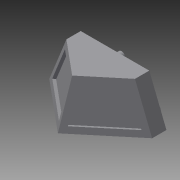
# Autodesk Inventor part: Cow Catcher
Saved by Autodesk Inventor 2015 (Build 190159000, 159)
## iProperties
Created: 2018-03-27
Part Number: Cow Catcher
Material: Generic
Document SubType Name: Modeling
Designer: Administrator
Density: 1 g/cm^3
Appearance: Default
Author: Administrator
Autodesk Inventor part; units mm, degrees
ref_plane "YZ Plane" through (0, 0, 0) normal (1, 0, 0) x (0, 1, 0)
ref_plane "XZ Plane" through (0, 0, 0) normal (0, 1, 0) x (-1, 0, 0)
ref_plane "XY Plane" through (0, 0, 0) normal (0, 0, 1) x (1, 0, 0)
sketch "Sketch1" plane through (0, 0, 0) normal (0, 1, 0) x (-1, 0, 0)
  line L0 (-3.711, -25.8637) -> (-3.711, -32.2137)
  line L1 (-3.711, -32.2137) -> (-49.431, -32.2137)
  line L2 (-49.431, -32.2137) -> (-49.431, -25.8637)
  line L3 (-3.711, -25.8637) -> (-26.571, -6.8137)
  line L4 (-26.571, -6.8137) -> (-49.431, -25.8637)
  point P0 (0, 0)
  dimension "d0" = 6.35
  dimension "d1" = 6.35
  dimension "d2" = 45.72
  dimension "d3" = 22.86
  dimension "d4" = 22.86
  dimension "d5" = 25.4
  constraints: 10 end point, 2 perpendicular
  measures "d0" distance of L0.start L0.end
  measures "d1" distance of L1.end L2.end
  measures "d2" distance of L0.end L1.end
  measures "d3" horizontal distance of L3.end L2.end
  measures "d4" horizontal distance of L0.start L3.end
  measures "d5" distance from line of L3.end L1
ref_plane "Work Plane2" through (0, 19.05, 0) normal (0, 1, 0) x (1, 0, 0)
sketch "Sketch2" plane through (0, 19.05, 0) normal (0, 1, 0) x (1, 0, 0)
  line L0 (41.811, 32.2137) -> (11.331, 32.2137)
  line L1 (11.331, 32.2137) -> (11.331, 25.8637)
  line L2 (11.331, 25.8637) -> (26.571, 13.1637)
  line L3 (26.571, 13.1637) -> (41.811, 25.8637)
  line L4 (41.811, 25.8637) -> (41.811, 32.2137)
  point P0 (0, 0)
  point P1 (26.571, 6.8137)
  dimension "d8" = 6.35
  dimension "d9" = 6.35
  dimension "d10" = 15.24
  dimension "d11" = 15.24
  dimension "d12" = 30.48
  dimension "d15" = 0
  constraints: 10 end point, 1 perpendicular, 1 vertical
  measures "d8" distance of L0.end L1.end
  measures "d9" distance of L3.end L0.start
  measures "d10" horizontal distance of L2.end L3.end
  measures "d11" horizontal distance of L1.end L2.end
  measures "d12" distance of L0.start L0.end
  measures "d15" horizontal distance of point (26.571, 6.814) L2.end
loft "Loft1" add profiles "Sketch1", "Sketch2"
shell "Shell1" thickness 2.54 removed faces 1 at (26.571, 0, -23.7471)
sketch "Sketch4" plane through (26.571, 0, -6.8137) normal (0.6201737, 0.2480695, 0.7442084) x (0.7682213, 0, -0.6401844)
  line L0 (0, 0) -> (4.0652, 19.6647) projected
  line L1 (29.7571, 0) -> (23.9032, 19.6647) projected
  line L2 (29.7571, 0) -> (0, 0) projected
  line L3 (23.9032, 19.6647) -> (4.0652, 19.6647) projected
  line L4 (3.1188, 2.54) -> (6.1338, 17.1247)
  line L5 (6.1338, 17.1247) -> (22.0092, 17.1247)
  line L6 (22.0092, 17.1247) -> (26.3508, 2.54)
  line L7 (26.3508, 2.54) -> (3.1188, 2.54)
  point P0 (-24.7744, 2.9212)
  dimension "d21" = 2.54
  dimension "d22" = 2.54
  dimension "d23" = 2.54
  dimension "d24" = 2.54
  constraints: 8 end point, 5 parallel, 1 horizontal
  measures "d21" distance between parallel lines of L2 L7
  measures "d22" distance between parallel lines of L0 L4
  measures "d23" distance between parallel lines of L3 L5
  measures "d24" distance between parallel lines of L1 L6
extrude "Extrusion2" cut sketch "Sketch4" against normal blind 1.27 contours L4 L5 L6 L7
sketch "Sketch5" plane through (3.711, 0, -25.8637) normal (-0.6201737, 0.2480695, 0.7442084) x (0.7682213, 0, 0.6401844)
  line L0 (29.7571, 0) -> (0, 0)
  line L1 (24.1888, 19.6583) -> (4.3507, 19.6583)
  line L2 (3.4063, 2.54) -> (7.746, 17.1183)
  line L3 (7.746, 17.1183) -> (23.6246, 17.1183)
  line L4 (23.6246, 17.1183) -> (26.6383, 2.54)
  line L5 (26.6383, 2.54) -> (3.4063, 2.54)
  line L6 (0, 0) -> (5.8538, 19.6647) projected
  line L7 (29.7571, 0) -> (25.6919, 19.6647) projected
  point P0 (13.7067, -5.5182)
  point P1 (-24.7744, 2.9212)
  dimension "d27" = 2.54
  dimension "d29" = 2.54
  dimension "d32" = 2.54
  dimension "d34" = 2.54
  constraints: 12 end point, 4 parallel, 1 horizontal
  measures "d27" distance between parallel lines of L0 L5
  measures "d29" distance between parallel lines of L1 L3
  measures "d32" distance between parallel lines of L6 L2
  measures "d34" distance between parallel lines of L7 L4
extrude "Extrusion3" cut sketch "Sketch5" against normal blind 1.27
sketch "Sketch6" plane through (49.431, 0, -32.2137) normal (0, 0, -1) x (-1, 0, 0)
  circle A0 centre (6.985, 3.175) radius 1.5875
  circle A1 centre (22.86, 15.875) radius 1.5875
  circle A2 centre (38.735, 3.175) radius 1.5875
  line L0 (0, 0) -> (7.62, 19.05) projected
  line L1 (45.72, 0) -> (0, 0) projected
  line L2 (45.72, 0) -> (38.1, 19.05) projected
  line L3 (38.1, 19.05) -> (7.62, 19.05) projected
  point P0 (49.431, 0)
  dimension "d37" = 6.985
  dimension "d38" = 6.985
  dimension "d39" = 3.175
  dimension "d40" = 3.175
  dimension "d41" = 3.175
  dimension "d42" = 22.86
  dimension "d43" = 3.175
  dimension "d44" = 3.175
  dimension "d45" = 3.175
  constraints: 3 centre point
  measures "d37" horizontal distance of A0.centre L0.start
  measures "d38" horizontal distance of L1.start A2.centre
  measures "d39" distance from line of L1 A0.centre
  measures "d40" distance from line of L1 A2.centre
  measures "d41" distance from line of L3 A1.centre
  measures "d42" horizontal distance of L1.start A1.centre
  measures "d43" diameter of A1
  measures "d44" diameter of A2
  measures "d45" diameter of A0
extrude "Extrusion4" add sketch "Sketch6" along normal blind 3.175 contours A0 | A1 | A2
chamfer "Chamfer1" distance 0.254 angle 45 3 edges at (44.0335, 3.175, -35.3887) (28.1585, 15.875, -35.3887) (12.2835, 3.175, -35.3887)
body "Solid2"
